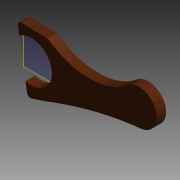
# Autodesk Inventor part: body01
Saved by Autodesk Inventor 2013 (Build 170138000, 138)
## iProperties
Created: 2013-02-19
Part Number: body01
Material: Wood (Walnut)
Document SubType Name: Modeling
Designer: Nano
Density: 0.55 g/cm^3
Mass: 9079.15 g
Surface Area: 6785.14 cm^2
Volume: 16507.6 cm^3
Author: Nano
Autodesk Inventor part; units mm, degrees
ref_plane "YZ Plane" through (0, 0, 0) normal (1, 0, 0) x (0, 1, 0)
ref_plane "XZ Plane" through (0, 0, 0) normal (0, 1, 0) x (-1, 0, 0)
ref_plane "XY Plane" through (0, 0, 0) normal (0, 0, 1) x (1, 0, 0)
ref_plane "Work Plane1" through (0, 0, -22.225) normal (0, 0, -1) x (-1, 0, 0)
sketch "Sketch1" plane through (0, 0, -22.225) normal (0, 0, -1) x (-1, 0, 0)
  arc A0 (88.9626, 123.799) -> (43.8693, -146.1511) centre (0.2092, -0.1167) ccw
  line L0 (104.0584, 214.2592) -> (-123.3104, 207.8545)
  line L1 (104.0584, 214.2592) -> (88.9626, 123.799)
  line L2 (27.3448, -245.173) -> (43.8693, -146.1511)
  spline S0 degree 3 poles (-707.521, 203.2816) (-551.4212, 75.7942) (-311.6817, 71.3053) (-123.3104, 207.8545) knots 0 0 0 0 1 1 1 1
  spline S1 degree 3 poles (-813.9039, -23.98) (-633.7548, -41.4595) (-396.5973, -89.7928) (-98.6304, -203.95) knots 0 0 0 0 1 1 1 1
  line L3 (-98.6304, -203.95) -> (27.3448, -245.173)
  arc A1 (-707.521, 203.2816) -> (-707.521, 203.2816) centre (-797.0248, 106.6489) ccw
  arc A2 (-707.521, 203.2816) -> (-707.521, 203.2816) centre (-797.0248, 106.6489) ccw
  line L4 (-754.135, 241.3513) -> (-660.9071, 165.2118) construction
  arc A3 (-742.7948, 235.6914) -> (-668.7183, 175.1928) centre (-447.3536, 521.8394) ccw construction
  line L5 (-880.3002, -17.5377) -> (-747.5076, -30.4223) construction
  arc A4 (-760.8772, -29.8585) -> (-867.0716, -19.5547) centre (-1002.1885, -1964.5023) ccw construction
  arc A5 (-707.521, 203.2816) -> (-806.8203, -24.6803) centre (-797.0248, 106.6609) ccw
  point P0 (-439.1346, 106.6934)
  point P1 (-549.9721, -66.3389)
  constraints: 13 end point, 6 point on circle, 4 centre point, 4 midpoint, 24 other
extrude "Extrusion1" add sketch "Sketch1" against normal blind 69.85 contours A0 L2 L3 S1 A1 S0 L0 L1 | A1 S1 A5 | A1 A5 | A5 S1 A1 | A5 S1 picked at (-815.5268, 64.2979) picked at (-885.3981, 33.5572)
fillet "Fillet1" radius 25.4 1 edges at (-104.0584, 214.2592, 12.7)
fillet "Fillet2" radius 25.4 1 edges at (-27.3448, -245.173, 12.7)
fillet "Fillet3" [suppressed]
body "Solid1"
